Autodesk Inventor part; units mm, degrees
(part 4 of 6)
  spline S23 degree 3 poles (-75.895, -170.0979) (-76.003, -170.1756) (-76.0512, -170.2099) (-76.1511, -170.2771) (-77.0955, -170.9125) (-78.4258, -171.5509) (-78.1911, -172.9231) (-77.9322, -174.437) (-76.2319, -174.5829) (-75.0125, -174.8445) (-74.2668, -175.0044) (-73.5211, -175.1644) (-72.7754, -175.3243) (-72.271, -175.4325) (-71.2647, -175.4898) (-70.9411, -175.9493) (-70.2467, -176.9353) (-72.2132, -178.4228) (-72.7983, -178.9937) (-74.0354, -180.2009) (-75.4699, -181.3587) (-76.535, -182.7209) (-77.4692, -183.9159) (-77.7659, -185.5032) (-76.3654, -186.4583) (-75.4147, -187.1067) (-74.3957, -185.8674) (-74.8747, -184.9677) (-75.0528, -184.6332) (-74.2251, -183.9061) (-74.0338, -183.712) (-73.3913, -183.0602) (-72.742, -182.4152) (-72.0961, -181.7668) (-71.0225, -180.689) (-69.6734, -179.6232) (-68.924, -178.2762) (-68.2015, -176.9778) (-68.162, -175.2179) (-69.3032, -174.1373) (-70.3851, -173.1128) (-72.1255, -172.999) (-73.5121, -172.7078) (-73.9141, -172.6234) (-74.3161, -172.5389) (-74.7181, -172.4545) (-74.8048, -172.4363) (-74.959, -172.3873) (-75.1286, -172.3366) knots 2.88117 2.88117 2.88117 2.88117 3 3 3 4 4 4 5 5 5 6 6 6 7 7 7 8 8 8 9 9 9 10 10 10 11 11 11 12 12 12 13 13 13 14 14 14 15 15 15 16 16 16 17 17 17 17.368094 17.368094 17.368094 17.368094
  line L312 (-75.895, -170.0979) -> (-76.003, -170.1756) construction
  line L313 (-76.003, -170.1756) -> (-76.0512, -170.2099) construction
  line L314 (-76.0512, -170.2099) -> (-76.1511, -170.2771) construction
  line L315 (-76.1511, -170.2771) -> (-77.0955, -170.9125) construction
  line L316 (-77.0955, -170.9125) -> (-78.4258, -171.5509) construction
  line L317 (-78.4258, -171.5509) -> (-78.1911, -172.9231) construction
  line L318 (-78.1911, -172.9231) -> (-77.9322, -174.437) construction
  line L319 (-77.9322, -174.437) -> (-76.2319, -174.5829) construction
  line L320 (-76.2319, -174.5829) -> (-75.0125, -174.8445) construction
  line L321 (-75.0125, -174.8445) -> (-74.2668, -175.0044) construction
  line L322 (-74.2668, -175.0044) -> (-73.5211, -175.1644) construction
  line L323 (-73.5211, -175.1644) -> (-72.7754, -175.3243) construction
  line L324 (-72.7754, -175.3243) -> (-72.271, -175.4325) construction
  line L325 (-72.271, -175.4325) -> (-71.2647, -175.4898) construction
  line L326 (-71.2647, -175.4898) -> (-70.9411, -175.9493) construction
  line L327 (-70.9411, -175.9493) -> (-70.2467, -176.9353) construction
  line L328 (-70.2467, -176.9353) -> (-72.2132, -178.4228) construction
  line L329 (-72.2132, -178.4228) -> (-72.7983, -178.9937) construction
  line L330 (-72.7983, -178.9937) -> (-74.0354, -180.2009) construction
  line L331 (-74.0354, -180.2009) -> (-75.4699, -181.3587) construction
  line L332 (-75.4699, -181.3587) -> (-76.535, -182.7209) construction
  line L333 (-76.535, -182.7209) -> (-77.4692, -183.9159) construction
  line L334 (-77.4692, -183.9159) -> (-77.7659, -185.5032) construction
  line L335 (-77.7659, -185.5032) -> (-76.3654, -186.4583) construction
  line L336 (-76.3654, -186.4583) -> (-75.4147, -187.1067) construction
  line L337 (-75.4147, -187.1067) -> (-74.3957, -185.8674) construction
  line L338 (-74.3957, -185.8674) -> (-74.8747, -184.9677) construction
  line L339 (-75.0528, -184.6332) -> (-74.2251, -183.9061) construction
  line L340 (-74.2251, -183.9061) -> (-74.0338, -183.712) construction
  line L341 (-74.0338, -183.712) -> (-73.3913, -183.0602) construction
  line L342 (-73.3913, -183.0602) -> (-72.742, -182.4152) construction
  line L343 (-72.742, -182.4152) -> (-72.0961, -181.7668) construction
  line L344 (-72.0961, -181.7668) -> (-71.0225, -180.689) construction
  line L345 (-71.0225, -180.689) -> (-69.6734, -179.6232) construction
  line L346 (-69.6734, -179.6232) -> (-68.924, -178.2762) construction
  line L347 (-68.924, -178.2762) -> (-68.2015, -176.9778) construction
  line L348 (-68.2015, -176.9778) -> (-68.162, -175.2179) construction
  line L349 (-68.162, -175.2179) -> (-69.3032, -174.1373) construction
  line L350 (-69.3032, -174.1373) -> (-70.3851, -173.1128) construction
  line L351 (-70.3851, -173.1128) -> (-72.1255, -172.999) construction
  line L352 (-72.1255, -172.999) -> (-73.5121, -172.7078) construction
  line L353 (-73.5121, -172.7078) -> (-73.9141, -172.6234) construction
  line L354 (-73.9141, -172.6234) -> (-74.3161, -172.5389) construction
  line L355 (-74.3161, -172.5389) -> (-74.7181, -172.4545) construction
  line L356 (-74.7181, -172.4545) -> (-74.8048, -172.4363) construction
  line L357 (-74.8048, -172.4363) -> (-74.959, -172.3873) construction
  line L358 (-74.959, -172.3873) -> (-75.1286, -172.3366) construction
  line L359 (-66.9691, -180.1793) -> (-67.2323, -182.0243) construction
  spline S24 degree 3 poles (-66.3184, -172.1966) (-66.3889, -173.6221) (-66.49, -175.0458) (-66.6098, -176.468) (-66.7663, -178.3251) (-66.9691, -180.1793) (-67.2323, -182.0243) (-67.498, -183.8869) (-67.9134, -185.8013) (-67.8984, -187.6872) (-67.8886, -188.9348) (-66.2915, -188.9842) (-65.8678, -187.962) (-64.8454, -185.4954) (-64.6389, -182.6096) (-64.3208, -179.9803) (-64.0008, -177.335) (-63.7894, -174.6802) (-63.6927, -172.0174) (-63.6735, -171.4906) (-63.6554, -170.9633) (-63.6452, -170.4361) knots 5.14687 5.14687 5.14687 5.14687 6 6 6 7 7 7 8 8 8 9 9 9 10 10 10 11 11 11 11.773986 11.773986 11.773986 11.773986
  line L360 (-66.3184, -172.1966) -> (-66.3889, -173.6221) construction
  line L361 (-66.3889, -173.6221) -> (-66.49, -175.0458) construction
  line L362 (-66.49, -175.0458) -> (-66.6098, -176.468) construction
  line L363 (-66.6098, -176.468) -> (-66.7663, -178.3251) construction
  line L364 (-66.7663, -178.3251) -> (-66.9691, -180.1793) construction
  line L365 (-67.2323, -182.0243) -> (-67.498, -183.8869) construction
  line L366 (-67.498, -183.8869) -> (-67.9134, -185.8013) construction
  line L367 (-67.9134, -185.8013) -> (-67.8984, -187.6872) construction
  line L368 (-67.8984, -187.6872) -> (-67.8886, -188.9348) construction
  line L369 (-67.8886, -188.9348) -> (-66.2915, -188.9842) construction
  line L370 (-66.2915, -188.9842) -> (-65.8678, -187.962) construction
  line L371 (-65.8678, -187.962) -> (-64.8454, -185.4954) construction
  line L372 (-64.8454, -185.4954) -> (-64.6389, -182.6096) construction
  line L373 (-64.6389, -182.6096) -> (-64.3208, -179.9803) construction
  line L374 (-64.3208, -179.9803) -> (-64.0008, -177.335) construction
  line L375 (-64.0008, -177.335) -> (-63.7894, -174.6802) construction
  line L376 (-63.7894, -174.6802) -> (-63.6927, -172.0174) construction
  line L377 (-63.6927, -172.0174) -> (-63.6735, -171.4906) construction
  line L378 (-63.6735, -171.4906) -> (-63.6554, -170.9633) construction
  line L379 (-63.6554, -170.9633) -> (-63.6452, -170.4361) construction
  line L380 (-72.2239, -170.1902) -> (-70.2415, -171.6221) construction
  spline S25 degree 3 poles (-70.3306, -165.8586) (-72.2715, -167.3246) (-72.2239, -170.1902) (-70.2415, -171.6221) (-69.0436, -172.4872) (-67.6209, -172.5969) (-66.3184, -172.1966) knots 0 0 0 0 1 1 1 1.551759 1.551759 1.551759 1.551759
  line L381 (-70.3306, -165.8586) -> (-72.2715, -167.3246) construction
  line L382 (-72.2715, -167.3246) -> (-72.2239, -170.1902) construction
  line L383 (-70.2415, -171.6221) -> (-69.0436, -172.4872) construction
  line L384 (-69.0436, -172.4872) -> (-67.6209, -172.5969) construction
  line L385 (-67.6209, -172.5969) -> (-66.3184, -172.1966) construction
  line L386 (-75.8438, -177.215) -> (-75.8598, -176.9127) construction
  spline S26 degree 3 poles (-75.8438, -177.215) (-75.8598, -176.9127) (-75.8749, -176.6103) (-75.8903, -176.308) knots 9 9 9 9 10 10 10 10
  line L387 (-75.8598, -176.9127) -> (-75.8749, -176.6103) construction
  line L388 (-75.8749, -176.6103) -> (-75.8903, -176.308) construction
  line L389 (-75.7872, -177.652) -> (-75.7991, -177.511) construction
  spline S27 degree 3 poles (-75.7872, -177.652) (-75.7991, -177.511) (-75.8388, -177.3089) (-75.8438, -177.215) knots 8.458233 8.458233 8.458233 8.458233 9 9 9 9
  line L390 (-75.7991, -177.511) -> (-75.8388, -177.3089) construction
  line L391 (-75.8388, -177.3089) -> (-75.8438, -177.215) construction
  line L392 (-75.8903, -176.308) -> (-75.9182, -175.7571) construction
  spline S28 degree 3 poles (-75.8903, -176.308) (-75.9182, -175.7571) (-75.9405, -175.2067) (-75.9478, -174.6554) knots 10 10 10 10 10.82684 10.82684 10.82684 10.82684
  line L393 (-75.9182, -175.7571) -> (-75.9405, -175.2067) construction
  line L394 (-75.9405, -175.2067) -> (-75.9478, -174.6554) construction
  line L395 (-75.1286, -172.3366) -> (-74.875, -172.1555) construction
  spline S29 degree 3 poles (-75.1286, -172.3366) (-74.875, -172.1555) (-74.6262, -171.9673) (-74.3834, -171.7721) (-73.31, -170.9091) (-71.8725, -169.6925) (-71.4682, -168.3217) (-70.528, -165.1341) (-74.6936, -164.6256) (-76.8233, -164.8814) (-80.0133, -165.2647) (-83.1726, -166.7988) (-85.2381, -169.2946) (-86.0068, -170.2234) (-84.7854, -171.5133) (-83.8916, -170.6411) knots 21.261625 21.261625 21.261625 21.261625 22 22 22 23 23 23 24 24 24 25 25 25 26 26 26 26
  line L396 (-74.875, -172.1555) -> (-74.6262, -171.9673) construction
  line L397 (-74.6262, -171.9673) -> (-74.3834, -171.7721) construction
  line L398 (-74.3834, -171.7721) -> (-73.31, -170.9091) construction
  line L399 (-73.31, -170.9091) -> (-71.8725, -169.6925) construction
  line L400 (-71.8725, -169.6925) -> (-71.4682, -168.3217) construction
  line L401 (-71.4682, -168.3217) -> (-70.528, -165.1341) construction
  line L402 (-70.528, -165.1341) -> (-74.6936, -164.6256) construction
  line L403 (-74.6936, -164.6256) -> (-76.8233, -164.8814) construction
  line L404 (-76.8233, -164.8814) -> (-80.0133, -165.2647) construction
  line L405 (-80.0133, -165.2647) -> (-83.1726, -166.7988) construction
  line L406 (-83.1726, -166.7988) -> (-85.2381, -169.2946) construction
  line L407 (-85.2381, -169.2946) -> (-86.0068, -170.2234) construction
  line L408 (-86.0068, -170.2234) -> (-84.7854, -171.5133) construction
  line L409 (-84.7854, -171.5133) -> (-83.8916, -170.6411) construction
  line L410 (-75.0942, -169.5218) -> (-75.895, -170.0979) construction
  spline S30 degree 3 poles (-83.8916, -170.6411) (-81.9705, -168.7663) (-79.6542, -167.4539) (-76.9735, -167.0639) (-76.2315, -166.956) (-74.1586, -166.6168) (-73.6261, -167.4082) (-73.2026, -168.0376) (-75.0942, -169.5218) (-75.895, -170.0979) knots 0 0 0 0 1 1 1 2 2 2 2.88117 2.88117 2.88117 2.88117
  line L411 (-83.8916, -170.6411) -> (-81.9705, -168.7663) construction
  line L412 (-81.9705, -168.7663) -> (-79.6542, -167.4539) construction
  line L413 (-79.6542, -167.4539) -> (-76.9735, -167.0639) construction
  line L414 (-76.9735, -167.0639) -> (-76.2315, -166.956) construction
  line L415 (-76.2315, -166.956) -> (-74.1586, -166.6168) construction
  line L416 (-74.1586, -166.6168) -> (-73.6261, -167.4082) construction
  line L417 (-73.6261, -167.4082) -> (-73.2026, -168.0376) construction
  line L418 (-73.2026, -168.0376) -> (-75.0942, -169.5218) construction
  line L419 (-63.5927, -170.3745) -> (-63.567, -170.3432) construction
  spline S31 degree 3 poles (-63.6452, -170.4361) (-63.6188, -170.4054) (-63.5927, -170.3745) (-63.567, -170.3432) (-62.7867, -169.3969) (-61.9982, -168.0447) (-62.8062, -166.8751) (-63.5854, -165.7473) (-65.1814, -165.8885) (-65.8312, -167.056) (-66.2446, -167.7987) (-66.3005, -168.7868) (-66.2949, -169.7471) knots 1.983848 1.983848 1.983848 1.983848 2 2 2 3 3 3 4 4 4 4.613609 4.613609 4.613609 4.613609
  line L420 (-63.6452, -170.4361) -> (-63.6188, -170.4054) construction
  line L421 (-63.6188, -170.4054) -> (-63.5927, -170.3745) construction
  line L422 (-63.567, -170.3432) -> (-62.7867, -169.3969) construction
  line L423 (-62.7867, -169.3969) -> (-61.9982, -168.0447) construction
  line L424 (-61.9982, -168.0447) -> (-62.8062, -166.8751) construction
  line L425 (-62.8062, -166.8751) -> (-63.5854, -165.7473) construction
  line L426 (-63.5854, -165.7473) -> (-65.1814, -165.8885) construction
  line L427 (-65.1814, -165.8885) -> (-65.8312, -167.056) construction
  line L428 (-65.8312, -167.056) -> (-66.2446, -167.7987) construction
  line L429 (-66.2446, -167.7987) -> (-66.3005, -168.7868) construction
  line L430 (-66.3005, -168.7868) -> (-66.2949, -169.7471) construction
  line L431 (-69.1768, -167.3539) -> (-68.3834, -166.6471) construction
  spline S32 degree 3 poles (-66.2949, -169.7471) (-66.4018, -169.8131) (-66.5128, -169.8731) (-66.6282, -169.926) (-67.4749, -170.3139) (-68.6499, -170.2541) (-69.3089, -169.5317) (-69.8927, -168.8917) (-69.801, -167.91) (-69.1768, -167.3539) (-68.3834, -166.6471) (-69.4605, -165.2013) (-70.3306, -165.8586) knots 16.74527 16.74527 16.74527 16.74527 17 17 17 18 18 18 19 19 19 20 20 20 20
  line L432 (-66.2949, -169.7471) -> (-66.4018, -169.8131) construction
  line L433 (-66.4018, -169.8131) -> (-66.5128, -169.8731) construction
  line L434 (-66.5128, -169.8731) -> (-66.6282, -169.926) construction
  line L435 (-66.6282, -169.926) -> (-67.4749, -170.3139) construction
  line L436 (-67.4749, -170.3139) -> (-68.6499, -170.2541) construction
  line L437 (-68.6499, -170.2541) -> (-69.3089, -169.5317) construction
  line L438 (-69.3089, -169.5317) -> (-69.8927, -168.8917) construction
  line L439 (-69.8927, -168.8917) -> (-69.801, -167.91) construction
  line L440 (-69.801, -167.91) -> (-69.1768, -167.3539) construction
  line L441 (-68.3834, -166.6471) -> (-69.4605, -165.2013) construction
  line L442 (-69.4605, -165.2013) -> (-70.3306, -165.8586) construction
  circle A2 centre (-64.2611, -168.0447) radius 0.8171
  line L443 (-63.026, -193.1432) -> (-63.7946, -194.072) construction
  spline S33 degree 3 poles (-52.9165, -196.1852) (-52.6628, -196.0041) (-52.4141, -195.8159) (-52.1712, -195.6207) (-51.0979, -194.7577) (-49.6604, -193.5411) (-49.256, -192.1703) (-48.3158, -188.9827) (-52.4814, -188.4742) (-54.6112, -188.7301) (-57.8011, -189.1133) (-60.9605, -190.6474) (-63.026, -193.1432) (-63.7946, -194.072) (-62.5732, -195.3619) (-61.6795, -194.4897) knots 21.261625 21.261625 21.261625 21.261625 22 22 22 23 23 23 24 24 24 25 25 25 26 26 26 26
  line L444 (-52.9165, -196.1852) -> (-52.6628, -196.0041) construction
  line L445 (-52.6628, -196.0041) -> (-52.4141, -195.8159) construction
  line L446 (-52.4141, -195.8159) -> (-52.1712, -195.6207) construction
  line L447 (-52.1712, -195.6207) -> (-51.0979, -194.7577) construction
  line L448 (-51.0979, -194.7577) -> (-49.6604, -193.5411) construction
  line L449 (-49.6604, -193.5411) -> (-49.256, -192.1703) construction
  line L450 (-49.256, -192.1703) -> (-48.3158, -188.9827) construction
  line L451 (-48.3158, -188.9827) -> (-52.4814, -188.4742) construction
  line L452 (-52.4814, -188.4742) -> (-54.6112, -188.7301) construction
  line L453 (-54.6112, -188.7301) -> (-57.8011, -189.1133) construction
  line L454 (-57.8011, -189.1133) -> (-60.9605, -190.6474) construction
  line L455 (-60.9605, -190.6474) -> (-63.026, -193.1432) construction
  line L456 (-63.7946, -194.072) -> (-62.5732, -195.3619) construction
  line L457 (-62.5732, -195.3619) -> (-61.6795, -194.4897) construction
  line L458 (-61.6795, -194.4897) -> (-59.7584, -192.6149) construction
  spline S34 degree 3 poles (-61.6795, -194.4897) (-59.7584, -192.6149) (-57.4421, -191.3025) (-54.7614, -190.9125) (-54.0194, -190.8046) (-51.9464, -190.4654) (-51.414, -191.2568) (-50.9905, -191.8862) (-52.882, -193.3704) (-53.6828, -193.9465) knots 0 0 0 0 1 1 1 2 2 2 2.88117 2.88117 2.88117 2.88117
  line L459 (-59.7584, -192.6149) -> (-57.4421, -191.3025) construction
  line L460 (-57.4421, -191.3025) -> (-54.7614, -190.9125) construction
  line L461 (-54.7614, -190.9125) -> (-54.0194, -190.8046) construction
  line L462 (-54.0194, -190.8046) -> (-51.9464, -190.4654) construction
  line L463 (-51.9464, -190.4654) -> (-51.414, -191.2568) construction
  line L464 (-51.414, -191.2568) -> (-50.9905, -191.8862) construction
  line L465 (-50.9905, -191.8862) -> (-52.882, -193.3704) construction
  line L466 (-52.882, -193.3704) -> (-53.6828, -193.9465) construction
  line L467 (-55.979, -196.7717) -> (-55.72, -198.2856) construction
  spline S35 degree 3 poles (-53.6828, -193.9465) (-53.7908, -194.0242) (-53.839, -194.0585) (-53.939, -194.1257) (-54.8833, -194.7611) (-56.2137, -195.3995) (-55.979, -196.7717) (-55.72, -198.2856) (-54.0197, -198.4315) (-52.8004, -198.6931) (-52.0547, -198.853) (-51.309, -199.013) (-50.5632, -199.1729) (-50.0588, -199.2811) (-49.0526, -199.3384) (-48.7289, -199.7979) (-48.0345, -200.7839) (-50.001, -202.2714) (-50.5861, -202.8424) (-51.8232, -204.0495) (-53.2578, -205.2073) (-54.3228, -206.5696) (-55.257, -207.7645) (-55.5537, -209.3518) (-54.1533, -210.3069) (-53.2025, -210.9553) (-52.1835, -209.716) (-52.6626, -208.8163) (-52.8407, -208.4818) (-52.0129, -207.7547) (-51.8216, -207.5606) (-51.1792, -206.9089) (-50.5298, -206.2638) (-49.884, -205.6154) (-48.8103, -204.5376) (-47.4613, -203.4718) (-46.7118, -202.1248) (-45.9894, -200.8264) (-45.9499, -199.0665) (-47.0911, -197.9859) (-48.173, -196.9614) (-49.9134, -196.8477) (-51.3, -196.5564) (-51.702, -196.472) (-52.104, -196.3875) (-52.506, -196.3031) (-52.5926, -196.2849) (-52.7469, -196.2359) (-52.9165, -196.1852) knots 2.88117 2.88117 2.88117 2.88117 3 3 3 4 4 4 5 5 5 6 6 6 7 7 7 8 8 8 9 9 9 10 10 10 11 11 11 12 12 12 13 13 13 14 14 14 15 15 15 16 16 16 17 17 17 17.368094 17.368094 17.368094 17.368094
  line L468 (-53.6828, -193.9465) -> (-53.7908, -194.0242) construction
  line L469 (-53.7908, -194.0242) -> (-53.839, -194.0585) construction
  line L470 (-53.839, -194.0585) -> (-53.939, -194.1257) construction
  line L471 (-53.939, -194.1257) -> (-54.8833, -194.7611) construction
  line L472 (-54.8833, -194.7611) -> (-56.2137, -195.3995) construction
  line L473 (-56.2137, -195.3995) -> (-55.979, -196.7717) construction
  line L474 (-55.72, -198.2856) -> (-54.0197, -198.4315) construction
  line L475 (-54.0197, -198.4315) -> (-52.8004, -198.6931) construction
  line L476 (-52.8004, -198.6931) -> (-52.0547, -198.853) construction
  line L477 (-52.0547, -198.853) -> (-51.309, -199.013) construction
  line L478 (-51.309, -199.013) -> (-50.5632, -199.1729) construction
  line L479 (-50.5632, -199.1729) -> (-50.0588, -199.2811) construction
  line L480 (-50.0588, -199.2811) -> (-49.0526, -199.3384) construction
  line L481 (-49.0526, -199.3384) -> (-48.7289, -199.7979) construction
  line L482 (-48.7289, -199.7979) -> (-48.0345, -200.7839) construction
  line L483 (-48.0345, -200.7839) -> (-50.001, -202.2714) construction
  line L484 (-50.001, -202.2714) -> (-50.5861, -202.8424) construction
  line L485 (-50.5861, -202.8424) -> (-51.8232, -204.0495) construction
  line L486 (-51.8232, -204.0495) -> (-53.2578, -205.2073) construction
  line L487 (-53.2578, -205.2073) -> (-54.3228, -206.5696) construction
  line L488 (-54.3228, -206.5696) -> (-55.257, -207.7645) construction
  line L489 (-55.257, -207.7645) -> (-55.5537, -209.3518) construction
  line L490 (-55.5537, -209.3518) -> (-54.1533, -210.3069) construction
  line L491 (-54.1533, -210.3069) -> (-53.2025, -210.9553) construction
  line L492 (-53.2025, -210.9553) -> (-52.1835, -209.716) construction
  line L493 (-52.1835, -209.716) -> (-52.6626, -208.8163) construction
  line L494 (-52.6626, -208.8163) -> (-52.8407, -208.4818) construction
  line L495 (-52.8407, -208.4818) -> (-52.0129, -207.7547) construction
  line L496 (-52.0129, -207.7547) -> (-51.8216, -207.5606) construction
  line L497 (-51.8216, -207.5606) -> (-51.1792, -206.9089) construction
  line L498 (-51.1792, -206.9089) -> (-50.5298, -206.2638) construction
  line L499 (-50.5298, -206.2638) -> (-49.884, -205.6154) construction
  line L500 (-49.884, -205.6154) -> (-48.8103, -204.5376) construction
  line L501 (-48.8103, -204.5376) -> (-47.4613, -203.4718) construction
  line L502 (-47.4613, -203.4718) -> (-46.7118, -202.1248) construction
  line L503 (-46.7118, -202.1248) -> (-45.9894, -200.8264) construction
  line L504 (-45.9894, -200.8264) -> (-45.9499, -199.0665) construction
  line L505 (-45.9499, -199.0665) -> (-47.0911, -197.9859) construction
  line L506 (-47.0911, -197.9859) -> (-48.173, -196.9614) construction
  line L507 (-48.173, -196.9614) -> (-49.9134, -196.8477) construction
  line L508 (-49.9134, -196.8477) -> (-51.3, -196.5564) construction
  line L509 (-51.3, -196.5564) -> (-51.702, -196.472) construction
  line L510 (-51.702, -196.472) -> (-52.104, -196.3875) construction
  line L511 (-52.104, -196.3875) -> (-52.506, -196.3031) construction
  line L512 (-52.506, -196.3031) -> (-52.5926, -196.2849) construction
  line L513 (-52.5926, -196.2849) -> (-52.7469, -196.2359) construction
  line L514 (-52.7469, -196.2359) -> (-52.9165, -196.1852) construction
  line L515 (-53.7283, -199.0553) -> (-53.7357, -198.504) construction
  spline S36 degree 3 poles (-53.6781, -200.1566) (-53.7061, -199.6057) (-53.7283, -199.0553) (-53.7357, -198.504) knots 10 10 10 10 10.82684 10.82684 10.82684 10.82684
  line L516 (-53.6781, -200.1566) -> (-53.7061, -199.6057) construction
  line L517 (-53.7061, -199.6057) -> (-53.7283, -199.0553) construction
  line L518 (-53.6628, -200.4589) -> (-53.6781, -200.1566) construction
  spline S37 degree 3 poles (-53.6316, -201.0636) (-53.6477, -200.7613) (-53.6628, -200.4589) (-53.6781, -200.1566) knots 9 9 9 9 10 10 10 10
  line L519 (-53.6316, -201.0636) -> (-53.6477, -200.7613) construction
  line L520 (-53.6477, -200.7613) -> (-53.6628, -200.4589) construction
  line L521 (-53.6266, -201.1575) -> (-53.6316, -201.0636) construction
  spline S38 degree 3 poles (-53.5751, -201.5006) (-53.5869, -201.3596) (-53.6266, -201.1575) (-53.6316, -201.0636) knots 8.458233 8.458233 8.458233 8.458233 9 9 9 9
  line L522 (-53.5751, -201.5006) -> (-53.5869, -201.3596) construction
  line L523 (-53.5869, -201.3596) -> (-53.6266, -201.1575) construction
  line L524 (-53.6828, -193.9465) -> (-53.8943, -193.0705) construction
  spline S39 degree 3 poles (-53.6828, -193.9465) (-53.8943, -193.0705) (-55.2251, -192.8666) (-55.5974, -193.9028) (-56.249, -195.7162) (-56.0849, -198.0729) (-55.9909, -199.975) (-55.9519, -200.7623) (-55.9989, -201.8724) (-55.5696, -202.5643) (-55.1597, -203.225) (-54.3745, -203.53) (-53.6994, -203.0943) (-53.1499, -202.7397) (-53.1315, -201.8791) (-53.5751, -201.5006) knots 1.141449 1.141449 1.141449 1.141449 2 2 2 3 3 3 4 4 4 5 5 5 5.747549 5.747549 5.747549 5.747549
  line L525 (-53.8943, -193.0705) -> (-55.2251, -192.8666) construction
  line L526 (-55.2251, -192.8666) -> (-55.5974, -193.9028) construction
  line L527 (-55.5974, -193.9028) -> (-56.249, -195.7162) construction
  line L528 (-56.249, -195.7162) -> (-56.0849, -198.0729) construction
  line L529 (-56.0849, -198.0729) -> (-55.9909, -199.975) construction
  line L530 (-55.9909, -199.975) -> (-55.9519, -200.7623) construction
  line L531 (-55.9519, -200.7623) -> (-55.9989, -201.8724) construction
  line L532 (-55.9989, -201.8724) -> (-55.5696, -202.5643) construction
  line L533 (-55.5696, -202.5643) -> (-55.1597, -203.225) construction
  line L534 (-55.1597, -203.225) -> (-54.3745, -203.53) construction
  line L535 (-54.3745, -203.53) -> (-53.6994, -203.0943) construction
  line L536 (-53.6994, -203.0943) -> (-53.1499, -202.7397) construction
  line L537 (-53.1499, -202.7397) -> (-53.1315, -201.8791) construction
  line L538 (-53.1315, -201.8791) -> (-53.5751, -201.5006) construction
  line L539 (-50.0118, -194.0388) -> (-48.0293, -195.4707) construction
  spline S40 degree 3 poles (-48.1185, -189.7072) (-50.0594, -191.1732) (-50.0118, -194.0388) (-48.0293, -195.4707) (-46.8315, -196.3358) (-45.4088, -196.4455) (-44.1063, -196.0452) knots 0 0 0 0 1 1 1 1.551759 1.551759 1.551759 1.551759
  line L540 (-48.1185, -189.7072) -> (-50.0594, -191.1732) construction
  line L541 (-50.0594, -191.1732) -> (-50.0118, -194.0388) construction
  line L542 (-48.0293, -195.4707) -> (-46.8315, -196.3358) construction
  line L543 (-46.8315, -196.3358) -> (-45.4088, -196.4455) construction
  line L544 (-45.4088, -196.4455) -> (-44.1063, -196.0452) construction
  line L545 (-46.4378, -194.1027) -> (-47.0968, -193.3803) construction
  spline S41 degree 3 poles (-44.0827, -193.5957) (-44.1897, -193.6617) (-44.3007, -193.7217) (-44.4161, -193.7746) (-45.2628, -194.1625) (-46.4378, -194.1027) (-47.0968, -193.3803) (-47.6806, -192.7403) (-47.5889, -191.7586) (-46.9647, -191.2026) (-46.1713, -190.4957) (-47.2483, -189.0499) (-48.1185, -189.7072) knots 16.74527 16.74527 16.74527 16.74527 17 17 17 18 18 18 19 19 19 20 20 20 20
  line L546 (-44.0827, -193.5957) -> (-44.1897, -193.6617) construction
  line L547 (-44.1897, -193.6617) -> (-44.3007, -193.7217) construction
  line L548 (-44.3007, -193.7217) -> (-44.4161, -193.7746) construction
  line L549 (-44.4161, -193.7746) -> (-45.2628, -194.1625) construction
  line L550 (-45.2628, -194.1625) -> (-46.4378, -194.1027) construction
  line L551 (-47.0968, -193.3803) -> (-47.6806, -192.7403) construction
  line L552 (-47.6806, -192.7403) -> (-47.5889, -191.7586) construction
  line L553 (-47.5889, -191.7586) -> (-46.9647, -191.2026) construction
  line L554 (-46.9647, -191.2026) -> (-46.1713, -190.4957) construction
  line L555 (-46.1713, -190.4957) -> (-47.2483, -189.0499) construction
  line L556 (-47.2483, -189.0499) -> (-48.1185, -189.7072) construction
  line L557 (-41.4432, -194.8119) -> (-41.4331, -194.2847) construction
  spline S42 degree 3 poles (-44.1063, -196.0452) (-44.1767, -197.4707) (-44.2779, -198.8944) (-44.3977, -200.3166) (-44.5541, -202.1737) (-44.757, -204.0279) (-45.0202, -205.8729) (-45.2859, -207.7355) (-45.7012, -209.6499) (-45.6863, -211.5358) (-45.6765, -212.7834) (-44.0793, -212.8328) (-43.6556, -211.8106) (-42.6332, -209.344) (-42.4267, -206.4582) (-42.1087, -203.8289) (-41.7887, -201.1836) (-41.5773, -198.5288) (-41.4805, -195.866) (-41.4614, -195.3392) (-41.4432, -194.8119) (-41.4331, -194.2847) knots 5.14687 5.14687 5.14687 5.14687 6 6 6 7 7 7 8 8 8 9 9 9 10 10 10 11 11 11 11.773986 11.773986 11.773986 11.773986
  line L558 (-44.1063, -196.0452) -> (-44.1767, -197.4707) construction
  line L559 (-44.1767, -197.4707) -> (-44.2779, -198.8944) construction
  line L560 (-44.2779, -198.8944) -> (-44.3977, -200.3166) construction
  line L561 (-44.3977, -200.3166) -> (-44.5541, -202.1737) construction
  line L562 (-44.5541, -202.1737) -> (-44.757, -204.0279) construction
  line L563 (-44.757, -204.0279) -> (-45.0202, -205.8729) construction
  line L564 (-45.0202, -205.8729) -> (-45.2859, -207.7355) construction
  line L565 (-45.2859, -207.7355) -> (-45.7012, -209.6499) construction
  line L566 (-45.7012, -209.6499) -> (-45.6863, -211.5358) construction
  line L567 (-45.6863, -211.5358) -> (-45.6765, -212.7834) construction
  line L568 (-45.6765, -212.7834) -> (-44.0793, -212.8328) construction
  line L569 (-44.0793, -212.8328) -> (-43.6556, -211.8106) construction
  line L570 (-43.6556, -211.8106) -> (-42.6332, -209.344) construction
  line L571 (-42.6332, -209.344) -> (-42.4267, -206.4582) construction
  line L572 (-42.4267, -206.4582) -> (-42.1087, -203.8289) construction
  line L573 (-42.1087, -203.8289) -> (-41.7887, -201.1836) construction
  line L574 (-41.7887, -201.1836) -> (-41.5773, -198.5288) construction
  line L575 (-41.5773, -198.5288) -> (-41.4805, -195.866) construction
  line L576 (-41.4805, -195.866) -> (-41.4614, -195.3392) construction
  line L577 (-41.4614, -195.3392) -> (-41.4432, -194.8119) construction
  line L578 (-41.3806, -194.2231) -> (-41.3548, -194.1918) construction
  spline S43 degree 3 poles (-41.4331, -194.2847) (-41.4067, -194.254) (-41.3806, -194.2231) (-41.3548, -194.1918) (-40.5746, -193.2455) (-39.7861, -191.8933) (-40.5941, -190.7237) (-41.3732, -189.5959) (-42.9692, -189.7371) (-43.6191, -190.9046) (-44.0325, -191.6473) (-44.0884, -192.6354) (-44.0827, -193.5957) knots 1.983848 1.983848 1.983848 1.983848 2 2 2 3 3 3 4 4 4 4.613609 4.613609 4.613609 4.613609
  line L579 (-41.4331, -194.2847) -> (-41.4067, -194.254) construction
  line L580 (-41.4067, -194.254) -> (-41.3806, -194.2231) construction
  line L581 (-41.3548, -194.1918) -> (-40.5746, -193.2455) construction
  line L582 (-40.5746, -193.2455) -> (-39.7861, -191.8933) construction
  line L583 (-39.7861, -191.8933) -> (-40.5941, -190.7237) construction
  line L584 (-40.5941, -190.7237) -> (-41.3732, -189.5959) construction
  line L585 (-41.3732, -189.5959) -> (-42.9692, -189.7371) construction
  line L586 (-42.9692, -189.7371) -> (-43.6191, -190.9046) construction
  line L587 (-43.6191, -190.9046) -> (-44.0325, -191.6473) construction
  line L588 (-44.0325, -191.6473) -> (-44.0884, -192.6354) construction
  line L589 (-44.0884, -192.6354) -> (-44.0827, -193.5957) construction
  circle A3 centre (-42.049, -191.8933) radius 0.8171
  line L590 (-92.0871, -183.9641) -> (-91.4831, -184.1987) construction
  spline S44 degree 3 poles (-90.951, -176.8268) (-91.1137, -176.1529) (-92.1374, -175.9961) (-92.4238, -176.7932) (-92.925, -178.1881) (-92.7988, -180.001) (-92.7264, -181.4642) (-92.6965, -182.0697) (-92.7326, -182.9236) (-92.4024, -183.4559) (-92.0871, -183.9641) (-91.4831, -184.1987) (-90.9637, -183.8636) (-90.5411, -183.5908) (-90.5269, -182.9289) (-90.8681, -182.6377) knots 1.141449 1.141449 1.141449 1.141449 2 2 2 3 3 3 4 4 4 5 5 5 5.747549 5.747549 5.747549 5.747549
  line L591 (-90.951, -176.8268) -> (-91.1137, -176.1529) construction
  line L592 (-91.1137, -176.1529) -> (-92.1374, -175.9961) construction
  line L593 (-92.1374, -175.9961) -> (-92.4238, -176.7932) construction
  line L594 (-92.4238, -176.7932) -> (-92.925, -178.1881) construction
  line L595 (-92.925, -178.1881) -> (-92.7988, -180.001) construction
  line L596 (-92.7988, -180.001) -> (-92.7264, -181.4642) construction
  line L597 (-92.7264, -181.4642) -> (-92.6965, -182.0697) construction
  line L598 (-92.6965, -182.0697) -> (-92.7326, -182.9236) construction
  line L599 (-92.7326, -182.9236) -> (-92.4024, -183.4559) construction
  line L600 (-92.4024, -183.4559) -> (-92.0871, -183.9641) construction
  line L601 (-91.4831, -184.1987) -> (-90.9637, -183.8636) construction
  line L602 (-90.9637, -183.8636) -> (-90.5411, -183.5908) construction
  line L603 (-90.5411, -183.5908) -> (-90.5269, -182.9289) construction
  line L604 (-90.5269, -182.9289) -> (-90.8681, -182.6377) construction
  line L605 (-90.8681, -182.6377) -> (-90.8772, -182.5292) construction
  spline S45 degree 3 poles (-90.8681, -182.6377) (-90.8772, -182.5292) (-90.9078, -182.3737) (-90.9116, -182.3015) knots 8.458233 8.458233 8.458233 8.458233 9 9 9 9
  line L606 (-90.8772, -182.5292) -> (-90.9078, -182.3737) construction
  line L607 (-90.9078, -182.3737) -> (-90.9116, -182.3015) construction
  line L608 (-90.9116, -182.3015) -> (-90.924, -182.0689) construction
  spline S46 degree 3 poles (-90.9116, -182.3015) (-90.924, -182.0689) (-90.9356, -181.8364) (-90.9474, -181.6038) knots 9 9 9 9 10 10 10 10
  line L609 (-90.924, -182.0689) -> (-90.9356, -181.8364) construction
  line L610 (-90.9356, -181.8364) -> (-90.9474, -181.6038) construction
  line L611 (-86.1652, -184.154) -> (-85.5887, -183.1178) construction
  spline S47 degree 3 poles (-90.951, -176.8268) (-91.0341, -176.8866) (-91.0712, -176.913) (-91.148, -176.9647) (-91.8745, -177.4535) (-92.8978, -177.9445) (-92.7173, -179) (-92.5181, -180.1646) (-91.2102, -180.2768) (-90.2722, -180.478) (-89.6986, -180.6011) (-89.125, -180.7241) (-88.5513, -180.8472) (-88.1633, -180.9304) (-87.3893, -180.9744) (-87.1403, -181.3279) (-86.6062, -182.0864) (-88.1189, -183.2306) (-88.5689, -183.6698) (-89.5205, -184.5984) (-90.6241, -185.489) (-91.4433, -186.5369) (-92.1619, -187.456) (-92.3902, -188.6771) (-91.3129, -189.4118) (-90.5816, -189.9105) (-89.7977, -188.9572) (-90.1662, -188.2651) (-90.3032, -188.0078) (-89.6665, -187.4485) (-89.5193, -187.2992) (-89.0251, -186.7979) (-88.5256, -186.3016) (-88.0288, -185.8029) (-87.2029, -184.9738) (-86.1652, -184.154) (-85.5887, -183.1178) (-85.033, -182.119) (-85.0026, -180.7653) (-85.8804, -179.934) (-86.7126, -179.146) (-88.0514, -179.0585) (-89.1181, -178.8344) (-89.4273, -178.7695) (-89.7365, -178.7045) (-90.0458, -178.6396) (-90.1124, -178.6256) (-90.2311, -178.5879) (-90.3615, -178.5489) knots 2.88117 2.88117 2.88117 2.88117 3 3 3 4 4 4 5 5 5 6 6 6 7 7 7 8 8 8 9 9 9 10 10 10 11 11 11 12 12 12 13 13 13 14 14 14 15 15 15 16 16 16 17 17 17 17.368094 17.368094 17.368094 17.368094
  line L612 (-90.951, -176.8268) -> (-91.0341, -176.8866) construction
  line L613 (-91.0341, -176.8866) -> (-91.0712, -176.913) construction
  line L614 (-91.0712, -176.913) -> (-91.148, -176.9647) construction
  line L615 (-91.148, -176.9647) -> (-91.8745, -177.4535) construction
  line L616 (-91.8745, -177.4535) -> (-92.8978, -177.9445) construction
  line L617 (-92.8978, -177.9445) -> (-92.7173, -179) construction
  line L618 (-92.7173, -179) -> (-92.5181, -180.1646) construction
  line L619 (-92.5181, -180.1646) -> (-91.2102, -180.2768) construction
  line L620 (-91.2102, -180.2768) -> (-90.2722, -180.478) construction
  line L621 (-90.2722, -180.478) -> (-89.6986, -180.6011) construction
  line L622 (-89.6986, -180.6011) -> (-89.125, -180.7241) construction
  line L623 (-89.125, -180.7241) -> (-88.5513, -180.8472) construction
  line L624 (-88.5513, -180.8472) -> (-88.1633, -180.9304) construction
  line L625 (-88.1633, -180.9304) -> (-87.3893, -180.9744) construction
  line L626 (-87.3893, -180.9744) -> (-87.1403, -181.3279) construction
  line L627 (-87.1403, -181.3279) -> (-86.6062, -182.0864) construction
  line L628 (-86.6062, -182.0864) -> (-88.1189, -183.2306) construction
  line L629 (-88.1189, -183.2306) -> (-88.5689, -183.6698) construction
  line L630 (-88.5689, -183.6698) -> (-89.5205, -184.5984) construction
  line L631 (-89.5205, -184.5984) -> (-90.6241, -185.489) construction
  line L632 (-90.6241, -185.489) -> (-91.4433, -186.5369) construction
  line L633 (-91.4433, -186.5369) -> (-92.1619, -187.456) construction
  line L634 (-92.1619, -187.456) -> (-92.3902, -188.6771) construction
  line L635 (-92.3902, -188.6771) -> (-91.3129, -189.4118) construction
  line L636 (-91.3129, -189.4118) -> (-90.5816, -189.9105) construction
  line L637 (-90.5816, -189.9105) -> (-89.7977, -188.9572) construction
  line L638 (-89.7977, -188.9572) -> (-90.1662, -188.2651) construction
  line L639 (-90.1662, -188.2651) -> (-90.3032, -188.0078) construction
  line L640 (-90.3032, -188.0078) -> (-89.6665, -187.4485) construction
  line L641 (-89.6665, -187.4485) -> (-89.5193, -187.2992) construction
  line L642 (-89.5193, -187.2992) -> (-89.0251, -186.7979) construction
  line L643 (-89.0251, -186.7979) -> (-88.5256, -186.3016) construction
  line L644 (-88.5256, -186.3016) -> (-88.0288, -185.8029) construction
  line L645 (-88.0288, -185.8029) -> (-87.2029, -184.9738) construction
  line L646 (-87.2029, -184.9738) -> (-86.1652, -184.154) construction
  line L647 (-85.5887, -183.1178) -> (-85.033, -182.119) construction
  line L648 (-85.033, -182.119) -> (-85.0026, -180.7653) construction
  line L649 (-85.0026, -180.7653) -> (-85.8804, -179.934) construction
  line L650 (-85.8804, -179.934) -> (-86.7126, -179.146) construction
  line L651 (-86.7126, -179.146) -> (-88.0514, -179.0585) construction
  line L652 (-88.0514, -179.0585) -> (-89.1181, -178.8344) construction
  line L653 (-89.1181, -178.8344) -> (-89.4273, -178.7695) construction
  line L654 (-89.4273, -178.7695) -> (-89.7365, -178.7045) construction
  line L655 (-89.7365, -178.7045) -> (-90.0458, -178.6396) construction
  line L656 (-90.0458, -178.6396) -> (-90.1124, -178.6256) construction
  line L657 (-90.1124, -178.6256) -> (-90.2311, -178.5879) construction
  line L658 (-90.2311, -178.5879) -> (-90.3615, -178.5489) construction
  line L659 (-90.9474, -181.6038) -> (-90.9689, -181.1801) construction
  spline S48 degree 3 poles (-90.9474, -181.6038) (-90.9689, -181.1801) (-90.986, -180.7567) (-90.9917, -180.3326) knots 10 10 10 10 10.82684 10.82684 10.82684 10.82684
  line L660 (-90.9689, -181.1801) -> (-90.986, -180.7567) construction
  line L661 (-90.986, -180.7567) -> (-90.9917, -180.3326) construction
  line L662 (-83.7165, -180.6329) -> (-83.8086, -181.7269) construction
  spline S49 degree 3 poles (-83.5844, -178.4412) (-83.6386, -179.5377) (-83.7165, -180.6329) (-83.8086, -181.7269) (-83.9289, -183.1554) (-84.085, -184.5817) (-84.2874, -186.001) (-84.4918, -187.4337) (-84.8113, -188.9063) (-84.7998, -190.3571) (-84.7923, -191.3168) (-83.5637, -191.3548) (-83.2378, -190.5685) (-82.4513, -188.671) (-82.2925, -186.4512) (-82.0478, -184.4287) (-81.8017, -182.3938) (-81.6391, -180.3517) (-81.5646, -178.3033) (-81.5499, -177.8981) (-81.5359, -177.4925) (-81.5281, -177.087) knots 5.14687 5.14687 5.14687 5.14687 6 6 6 7 7 7 8 8 8 9 9 9 10 10 10 11 11 11 11.773986 11.773986 11.773986 11.773986
  line L663 (-83.5844, -178.4412) -> (-83.6386, -179.5377) construction
  line L664 (-83.6386, -179.5377) -> (-83.7165, -180.6329) construction
  line L665 (-83.8086, -181.7269) -> (-83.9289, -183.1554) construction
  line L666 (-83.9289, -183.1554) -> (-84.085, -184.5817) construction
  line L667 (-84.085, -184.5817) -> (-84.2874, -186.001) construction
  line L668 (-84.2874, -186.001) -> (-84.4918, -187.4337) construction
  line L669 (-84.4918, -187.4337) -> (-84.8113, -188.9063) construction
  line L670 (-84.8113, -188.9063) -> (-84.7998, -190.3571) construction
  line L671 (-84.7998, -190.3571) -> (-84.7923, -191.3168) construction
  line L672 (-84.7923, -191.3168) -> (-83.5637, -191.3548) construction
  line L673 (-83.5637, -191.3548) -> (-83.2378, -190.5685) construction
  line L674 (-83.2378, -190.5685) -> (-82.4513, -188.671) construction
  line L675 (-82.4513, -188.671) -> (-82.2925, -186.4512) construction
  line L676 (-82.2925, -186.4512) -> (-82.0478, -184.4287) construction
  line L677 (-82.0478, -184.4287) -> (-81.8017, -182.3938) construction
  line L678 (-81.8017, -182.3938) -> (-81.6391, -180.3517) construction
  line L679 (-81.6391, -180.3517) -> (-81.5646, -178.3033) construction
  line L680 (-81.5646, -178.3033) -> (-81.5499, -177.8981) construction
  line L681 (-81.5499, -177.8981) -> (-81.5359, -177.4925) construction
  line L682 (-81.5359, -177.4925) -> (-81.5281, -177.087) construction
  line L683 (-90.1664, -178.4096) -> (-89.975, -178.2648) construction
  spline S50 degree 3 poles (-90.3615, -178.5489) (-90.1664, -178.4096) (-89.975, -178.2648) (-89.7882, -178.1146) (-88.9626, -177.4509) (-87.8568, -176.515) (-87.5458, -175.4605) (-86.8225, -173.0085) (-90.0269, -172.6174) (-91.6651, -172.8142) (-94.1189, -173.109) (-96.5492, -174.2891) (-98.1381, -176.2089) (-98.7293, -176.9233) (-97.7898, -177.9156) (-97.1023, -177.2446) knots 21.261625 21.261625 21.261625 21.261625 22 22 22 23 23 23 24 24 24 25 25 25 26 26 26 26
  line L684 (-90.3615, -178.5489) -> (-90.1664, -178.4096) construction
  line L685 (-89.975, -178.2648) -> (-89.7882, -178.1146) construction
  line L686 (-89.7882, -178.1146) -> (-88.9626, -177.4509) construction
  line L687 (-88.9626, -177.4509) -> (-87.8568, -176.515) construction
  line L688 (-87.8568, -176.515) -> (-87.5458, -175.4605) construction
  line L689 (-87.5458, -175.4605) -> (-86.8225, -173.0085) construction
  line L690 (-86.8225, -173.0085) -> (-90.0269, -172.6174) construction
  line L691 (-90.0269, -172.6174) -> (-91.6651, -172.8142) construction
  line L692 (-91.6651, -172.8142) -> (-94.1189, -173.109) construction
  line L693 (-94.1189, -173.109) -> (-96.5492, -174.2891) construction
  line L694 (-96.5492, -174.2891) -> (-98.1381, -176.2089) construction
  line L695 (-98.1381, -176.2089) -> (-98.7293, -176.9233) construction
  line L696 (-98.7293, -176.9233) -> (-97.7898, -177.9156) construction
  line L697 (-97.7898, -177.9156) -> (-97.1023, -177.2446) construction
  line L698 (-89.6153, -174.1491) -> (-89.2057, -174.7578) construction
  spline S51 degree 3 poles (-97.1023, -177.2446) (-95.6245, -175.8025) (-93.8427, -174.793) (-91.7807, -174.493) (-91.2099, -174.4099) (-89.6153, -174.1491) (-89.2057, -174.7578) (-88.88, -175.242) (-90.335, -176.3836) (-90.951, -176.8268) knots 0 0 0 0 1 1 1 2 2 2 2.88117 2.88117 2.88117 2.88117
  line L699 (-97.1023, -177.2446) -> (-95.6245, -175.8025) construction
  line L700 (-95.6245, -175.8025) -> (-93.8427, -174.793) construction
  line L701 (-93.8427, -174.793) -> (-91.7807, -174.493) construction
  line L702 (-91.7807, -174.493) -> (-91.2099, -174.4099) construction
  line L703 (-91.2099, -174.4099) -> (-89.6153, -174.1491) construction
  line L704 (-89.2057, -174.7578) -> (-88.88, -175.242) construction
  line L705 (-88.88, -175.242) -> (-90.335, -176.3836) construction
  line L706 (-90.335, -176.3836) -> (-90.951, -176.8268) construction
  line L707 (-83.734, -176.6539) -> (-83.8228, -176.6946) construction
  spline S52 degree 3 poles (-83.5663, -176.557) (-83.6486, -176.6078) (-83.734, -176.6539) (-83.8228, -176.6946) (-84.4741, -176.993) (-85.3779, -176.947) (-85.8848, -176.3913) (-86.3339, -175.899) (-86.2634, -175.1438) (-85.7832, -174.7161) (-85.1729, -174.1724) (-86.0014, -173.0602) (-86.6707, -173.5658) knots 16.74527 16.74527 16.74527 16.74527 17 17 17 18 18 18 19 19 19 20 20 20 20
  line L708 (-83.5663, -176.557) -> (-83.6486, -176.6078) construction
  line L709 (-83.6486, -176.6078) -> (-83.734, -176.6539) construction
  line L710 (-83.8228, -176.6946) -> (-84.4741, -176.993) construction
  line L711 (-84.4741, -176.993) -> (-85.3779, -176.947) construction
  line L712 (-85.3779, -176.947) -> (-85.8848, -176.3913) construction
  line L713 (-85.8848, -176.3913) -> (-86.3339, -175.899) construction
  line L714 (-86.3339, -175.899) -> (-86.2634, -175.1438) construction
  line L715 (-86.2634, -175.1438) -> (-85.7832, -174.7161) construction
  line L716 (-85.7832, -174.7161) -> (-85.1729, -174.1724) construction
  line L717 (-85.1729, -174.1724) -> (-86.0014, -173.0602) construction
  line L718 (-86.0014, -173.0602) -> (-86.6707, -173.5658) construction
  line L719 (-86.6022, -177.9993) -> (-85.6808, -178.6648) construction
  spline S53 degree 3 poles (-86.6707, -173.5658) (-88.1638, -174.6935) (-88.1271, -176.8979) (-86.6022, -177.9993) (-85.6808, -178.6648) (-84.5864, -178.7491) (-83.5844, -178.4412) knots 0 0 0 0 1 1 1 1.551759 1.551759 1.551759 1.551759
  line L720 (-86.6707, -173.5658) -> (-88.1638, -174.6935) construction
  line L721 (-88.1638, -174.6935) -> (-88.1271, -176.8979) construction
  line L722 (-88.1271, -176.8979) -> (-86.6022, -177.9993) construction
  line L723 (-85.6808, -178.6648) -> (-84.5864, -178.7491) construction
  line L724 (-84.5864, -178.7491) -> (-83.5844, -178.4412) construction
  line L725 (-81.5281, -177.087) -> (-81.5078, -177.0634) construction
  spline S54 degree 3 poles (-81.5281, -177.087) (-81.5078, -177.0634) (-81.4877, -177.0396) (-81.4679, -177.0155) (-80.8678, -176.2876) (-80.2612, -175.2475) (-80.8827, -174.3478) (-81.4821, -173.4802) (-82.7098, -173.5888) (-83.2096, -174.4869) (-83.5277, -175.0582) (-83.5707, -175.8183) (-83.5663, -176.557) knots 1.983848 1.983848 1.983848 1.983848 2 2 2 3 3 3 4 4 4 4.613609 4.613609 4.613609 4.613609
  line L726 (-81.5078, -177.0634) -> (-81.4877, -177.0396) construction
  line L727 (-81.4877, -177.0396) -> (-81.4679, -177.0155) construction
  line L728 (-81.4679, -177.0155) -> (-80.8678, -176.2876) construction
  line L729 (-80.8678, -176.2876) -> (-80.2612, -175.2475) construction
  line L730 (-80.2612, -175.2475) -> (-80.8827, -174.3478) construction
  line L731 (-80.8827, -174.3478) -> (-81.4821, -173.4802) construction
  line L732 (-81.4821, -173.4802) -> (-82.7098, -173.5888) construction
  line L733 (-82.7098, -173.5888) -> (-83.2096, -174.4869) construction
  line L734 (-83.2096, -174.4869) -> (-83.5277, -175.0582) construction
  line L735 (-83.5277, -175.0582) -> (-83.5707, -175.8183) construction
  line L736 (-83.5707, -175.8183) -> (-83.5663, -176.557) construction
  circle A4 centre (-82.0019, -175.2475) radius 0.6286
  line L737 (-3.2487, -226.4949) -> (-2.6446, -226.7295) construction
  spline S55 degree 3 poles (-2.1126, -219.3576) (-2.2752, -218.6837) (-3.2989, -218.5269) (-3.5853, -219.324) (-4.0865, -220.7189) (-3.9604, -222.5317) (-3.888, -223.9949) (-3.8581, -224.6005) (-3.8942, -225.4544) (-3.564, -225.9867) (-3.2487, -226.4949) (-2.6446, -226.7295) (-2.1253, -226.3944) (-1.7026, -226.1216) (-1.6885, -225.4596) (-2.0297, -225.1684) knots 1.141449 1.141449 1.141449 1.141449 2 2 2 3 3 3 4 4 4 5 5 5 5.747549 5.747549 5.747549 5.747549
  line L738 (-2.1126, -219.3576) -> (-2.2752, -218.6837) construction
  line L739 (-2.2752, -218.6837) -> (-3.2989, -218.5269) construction
  line L740 (-3.2989, -218.5269) -> (-3.5853, -219.324) construction
  line L741 (-3.5853, -219.324) -> (-4.0865, -220.7189) construction
  line L742 (-4.0865, -220.7189) -> (-3.9604, -222.5317) construction
  line L743 (-3.9604, -222.5317) -> (-3.888, -223.9949) construction
  line L744 (-3.888, -223.9949) -> (-3.8581, -224.6005) construction
  line L745 (-3.8581, -224.6005) -> (-3.8942, -225.4544) construction
  line L746 (-3.8942, -225.4544) -> (-3.564, -225.9867) construction
  line L747 (-3.564, -225.9867) -> (-3.2487, -226.4949) construction
  line L748 (-2.6446, -226.7295) -> (-2.1253, -226.3944) construction
  line L749 (-2.1253, -226.3944) -> (-1.7026, -226.1216) construction
  line L750 (-1.7026, -226.1216) -> (-1.6885, -225.4596) construction
  line L751 (-1.6885, -225.4596) -> (-2.0297, -225.1684) construction
  line L752 (2.6732, -226.6847) -> (3.2497, -225.6486) construction
  spline S56 degree 3 poles (-2.1126, -219.3576) (-2.1957, -219.4174) (-2.2328, -219.4438) (-2.3096, -219.4955) (-3.036, -219.9842) (-4.0594, -220.4753) (-3.8788, -221.5308) (-3.6797, -222.6954) (-2.3718, -222.8076) (-1.4338, -223.0088) (-0.8602, -223.1319) (-0.2865, -223.2549) (0.2871, -223.3779) (0.6751, -223.4612) (1.4491, -223.5052) (1.6981, -223.8587) (2.2322, -224.6172) (0.7196, -225.7614) (0.2695, -226.2006) (-0.6821, -227.1292) (-1.7856, -228.0198) (-2.6049, -229.0676) (-3.3235, -229.9868) (-3.5518, -231.2078) (-2.4745, -231.9425) (-1.7431, -232.4413) (-0.9593, -231.488) (-1.3278, -230.7959) (-1.4648, -230.5386) (-0.828, -229.9793) (-0.6809, -229.83) (-0.1867, -229.3286) (0.3128, -228.8324) (0.8096, -228.3337) (1.6355, -227.5046) (2.6732, -226.6847) (3.2497, -225.6486) (3.8054, -224.6498) (3.8358, -223.2961) (2.958, -222.4648) (2.1258, -221.6767) (0.787, -221.5893) (-0.2796, -221.3652) (-0.5889, -221.3003) (-0.8981, -221.2353) (-1.2073, -221.1704) (-1.274, -221.1564) (-1.3926, -221.1187) (-1.5231, -221.0797) knots 2.88117 2.88117 2.88117 2.88117 3 3 3 4 4 4 5 5 5 6 6 6 7 7 7 8 8 8 9 9 9 10 10 10 11 11 11 12 12 12 13 13 13 14 14 14 15 15 15 16 16 16 17 17 17 17.368094 17.368094 17.368094 17.368094
  line L753 (-2.1126, -219.3576) -> (-2.1957, -219.4174) construction
  line L754 (-2.1957, -219.4174) -> (-2.2328, -219.4438) construction
  line L755 (-2.2328, -219.4438) -> (-2.3096, -219.4955) construction
  line L756 (-2.3096, -219.4955) -> (-3.036, -219.9842) construction
  line L757 (-3.036, -219.9842) -> (-4.0594, -220.4753) construction
  line L758 (-4.0594, -220.4753) -> (-3.8788, -221.5308) construction
  line L759 (-3.8788, -221.5308) -> (-3.6797, -222.6954) construction
  line L760 (-3.6797, -222.6954) -> (-2.3718, -222.8076) construction
  line L761 (-2.3718, -222.8076) -> (-1.4338, -223.0088) construction
  line L762 (-1.4338, -223.0088) -> (-0.8602, -223.1319) construction
  line L763 (-0.8602, -223.1319) -> (-0.2865, -223.2549) construction
  line L764 (-0.2865, -223.2549) -> (0.2871, -223.3779) construction
  line L765 (0.2871, -223.3779) -> (0.6751, -223.4612) construction
  line L766 (0.6751, -223.4612) -> (1.4491, -223.5052) construction
  line L767 (1.4491, -223.5052) -> (1.6981, -223.8587) construction
  line L768 (1.6981, -223.8587) -> (2.2322, -224.6172) construction
  line L769 (2.2322, -224.6172) -> (0.7196, -225.7614) construction
  line L770 (0.7196, -225.7614) -> (0.2695, -226.2006) construction
  line L771 (0.2695, -226.2006) -> (-0.6821, -227.1292) construction
  line L772 (-0.6821, -227.1292) -> (-1.7856, -228.0198) construction
  line L773 (-1.7856, -228.0198) -> (-2.6049, -229.0676) construction
  line L774 (-2.6049, -229.0676) -> (-3.3235, -229.9868) construction
  line L775 (-3.3235, -229.9868) -> (-3.5518, -231.2078) construction
  line L776 (-3.5518, -231.2078) -> (-2.4745, -231.9425) construction
  line L777 (-2.4745, -231.9425) -> (-1.7431, -232.4413) construction
  line L778 (-1.7431, -232.4413) -> (-0.9593, -231.488) construction
  line L779 (-0.9593, -231.488) -> (-1.3278, -230.7959) construction
  line L780 (-1.3278, -230.7959) -> (-1.4648, -230.5386) construction
  line L781 (-1.4648, -230.5386) -> (-0.828, -229.9793) construction
  line L782 (-0.828, -229.9793) -> (-0.6809, -229.83) construction
  line L783 (-0.6809, -229.83) -> (-0.1867, -229.3286) construction
  line L784 (-0.1867, -229.3286) -> (0.3128, -228.8324) construction
  line L785 (0.3128, -228.8324) -> (0.8096, -228.3337) construction
  line L786 (0.8096, -228.3337) -> (1.6355, -227.5046) construction
  line L787 (1.6355, -227.5046) -> (2.6732, -226.6847) construction
  line L788 (3.2497, -225.6486) -> (3.8054, -224.6498) construction
  line L789 (3.8054, -224.6498) -> (3.8358, -223.2961) construction
  line L790 (3.8358, -223.2961) -> (2.958, -222.4648) construction
  line L791 (2.958, -222.4648) -> (2.1258, -221.6767) construction
  line L792 (2.1258, -221.6767) -> (0.787, -221.5893) construction
  line L793 (0.787, -221.5893) -> (-0.2796, -221.3652) construction
  line L794 (-0.2796, -221.3652) -> (-0.5889, -221.3003) construction
  line L795 (-0.5889, -221.3003) -> (-0.8981, -221.2353) construction